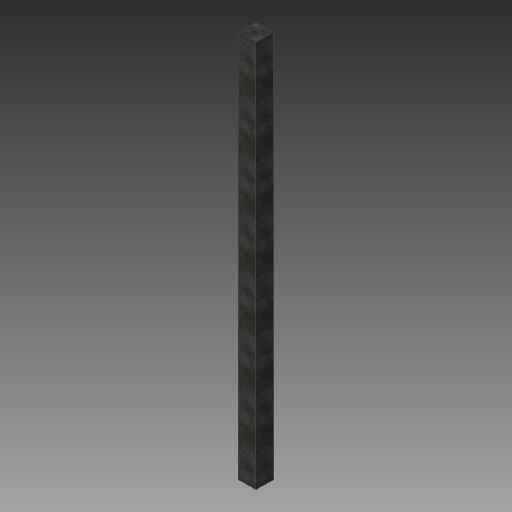
# Autodesk Inventor part: Cylinder
Saved by Autodesk Inventor 2017 (Build 210142000, 142)
## iProperties
Created: 2016-07-21
Part Number: Cylinder
Material: Steel
Document SubType Name: Modeling
Designer: Marcin
Density: 7.85 g/cm^3
Appearance: Plate
Mass: 32900.2 g
Surface Area: 4356.1 cm^2
Volume: 4191.1 cm^3
Author: Marcin
Autodesk Inventor part; units mm, degrees
ref_plane "YZ Plane" through (0, 0, 0) normal (1, 0, 0) x (0, 1, 0)
ref_plane "XZ Plane" through (0, 0, 0) normal (0, 1, 0) x (-1, 0, 0)
ref_plane "XY Plane" through (0, 0, 0) normal (0, 0, 1) x (1, 0, 0)
sketch "Sketch1" plane through (0, 0, 0) normal (0, 1, 0) x (-1, 0, 0)
  line L0 (-30, -30) -> (30, -30)
  line L1 (30, -30) -> (30, 30)
  line L2 (30, 30) -> (-30, 30)
  line L3 (-30, 30) -> (-30, -30)
  line L4 (-30, -30) -> (30, 30) construction
  line L5 (30, -30) -> (-30, 30) construction
  circle A0 centre (0, 0) radius 12.5
  dimension "d0" = 60
  dimension "d1" = 60
  dimension "d2" = 25
  constraints: 12 end point, 2 midpoint, 2 parallel, 1 centre point, 1 coincident, 1 horizontal, 1 perpendicular
  measures "d0" distance of L2.end L1.end
  measures "d1" distance of L1.end L0.end
  measures "d2" diameter of A0
extrude "Extrusion1" add sketch "Sketch1" along normal blind 1348
body "Solid1"
